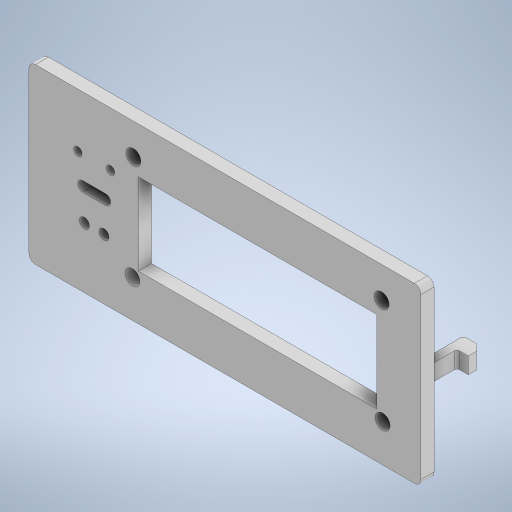
# Autodesk Inventor part: Front
Saved by Autodesk Inventor 2023 (Build 270158000, 158)
## iProperties
Created: 2023-01-08
Part Number: Front
Material: Generisch
Document SubType Name: Modeling
Designer: Benedikt
Density: 1 g/cm^3
Appearance: Vorgabe
Mass: 13.2 g
Surface Area: 108.904 cm^2
Volume: 13.2 cm^3
Author: Benedikt
Autodesk Inventor part; units mm, degrees
ref_plane "YZ Plane" through (0, 0, 0) normal (1, 0, 0) x (0, 1, 0)
ref_plane "XZ Plane" through (0, 0, 0) normal (0, 1, 0) x (-1, 0, 0)
ref_plane "XY Plane" through (0, 0, 0) normal (0, 0, 1) x (1, 0, 0)
sketch "Skizze1" plane through (0, 0, 0) normal (0, 0, 1) x (1, 0, 0)
  line L0 (-60, -26.5) -> (60, -26.5)
  line L1 (60, -26.5) -> (60, 26.5)
  line L2 (60, 26.5) -> (-60, 26.5)
  line L3 (-60, 26.5) -> (-60, -26.5)
  line L4 (-60, -26.5) -> (60, 26.5) construction
  line L5 (60, -26.5) -> (-60, 26.5) construction
  point P0 (0, 0)
  dimension "d0" = 53
  dimension "d1" = 120
  constraints: 12 end point, 2 midpoint, 2 parallel, 1 horizontal, 1 perpendicular
  measures "d0" distance of L0.end L1.end
  measures "d1" distance of L1.end L2.end
extrude "Extrusion1" add sketch "Skizze1" along normal blind 4
sketch "Skizze2" plane through (0, 0, 0) normal (0, 0, -1) x (-1, 0, 0)
  line L0 (-60, -23.5) -> (-60, -26.5) construction
  line L1 (-54, -4) -> (-56.5, -4)
  line L2 (-56.5, -4) -> (-56.5, 1)
  line L3 (-56.5, 1) -> (-54, 1)
  line L4 (-54, 1) -> (-54, -4)
  line L5 (-54, -4) -> (-56.5, 1) construction
  line L6 (-56.5, -4) -> (-54, 1) construction
  line L7 (54, -1) -> (56.5, -1)
  line L8 (56.5, -1) -> (56.5, 4)
  line L9 (56.5, 4) -> (54, 4)
  line L10 (54, 4) -> (54, -1)
  line L11 (54, -1) -> (56.5, 4) construction
  line L12 (56.5, -1) -> (54, 4) construction
  line L13 (60, -26.5) -> (-60, -26.5) projected
  point P0 (0, 0)
  point P1 (-55.25, -1.5)
  point P2 (-55.25, -1.5)
  dimension "d5" = 2.5
  dimension "d6" = 5
  dimension "d68" = 25
  constraints: 26 end point, 2 midpoint, 2 parallel, 1 horizontal, 1 perpendicular
  measures "d5" distance of L2.end L3.end
  measures "d6" distance of L3.end L1.start
  measures "d68" distance from line of L13 point (-55.25, -1.5)
extrude "Extrusion2" add sketch "Skizze2" along normal blind 15 contours L1 L2 L3 L4
sketch "Skizze6" plane through (56.5, -4, 0) normal (1, 0, 0) x (0, 0, -1)
  line L0 (15, 5) -> (15, 0) projected
  line L1 (15, 2.5) -> (0, 2.5)
  line L2 (0, -22.5) -> (0, 30.5) projected
  line L3 (10.5, 0) -> (15, 0)
  line L4 (15, 0) -> (15, 5)
  line L5 (15, 5) -> (10.5, 5)
  line L6 (10.5, 5) -> (10.5, 0)
  line L7 (10.5, 0) -> (15, 5) construction
  line L8 (15, 0) -> (10.5, 5) construction
  point P0 (0, 4)
  point P1 (12.75, 2.5)
  point P2 (15, 0)
  dimension "d19" = 4.5
  dimension "d20" = 5
  constraints: 14 end point, 3 midpoint, 3 point on line, 2 horizontal, 2 parallel, 1 perpendicular
  measures "d19" distance of L4.end L5.end
  measures "d20" distance of L5.end L3.start
extrude "Extrusion5" add sketch "Skizze6" along normal blind 3.5
mirror "Spiegeln2" about plane through (0, 0, 0) normal (1, 0, 0) of "Extrusion2", "Extrusion5"
sketch "Skizze7" plane through (0, 0, 4) normal (0, 0, 1) x (1, 0, 0)
  line L0 (-26.5, -12.5) -> (46.5, -12.5)
  line L1 (46.5, -12.5) -> (46.5, 12.5)
  line L2 (46.5, 12.5) -> (-26.5, 12.5)
  line L3 (-26.5, 12.5) -> (-26.5, -12.5)
  line L4 (-26.5, -12.5) -> (46.5, 12.5) construction
  line L5 (46.5, -12.5) -> (-26.5, 12.5) construction
  point P0 (0, 0)
  point P1 (10, 0)
  dimension "d23" = 10
  dimension "d24" = 73
  dimension "d25" = 25
  constraints: 12 end point, 2 midpoint, 2 parallel, 1 horizontal, 1 perpendicular
  measures "d23" distance of point (10, 0) point (0, 0)
  measures "d24" distance of L2.end L1.end
  measures "d25" distance of L1.end L0.end
extrude "Extrusion6" cut sketch "Skizze7" against normal through all
sketch "Skizze8" plane through (0, 0, 4) normal (0, 0, 1) x (1, 0, 0)
  line L0 (-60, 26.5) -> (-60, -26.5) projected
  line L1 (-60, 0) -> (60, 0)
  line L2 (60, -26.5) -> (60, 26.5) projected
  line L3 (-56, 10) -> (-26.5, 10) construction
  line L4 (-26.5, -12.5) -> (-26.5, 12.5) construction
  circle A0 centre (-45, 10) radius 1.25
  line L5 (-40, 10) -> (-40, 12.8313) construction
  circle A1 centre (-35, 10) radius 1.25
  line L6 (-40, 10) -> (-40, 0) construction
  line L7 (-43.5, 1.5) -> (-36.5, 1.5) construction
  line L8 (-43.5, 0) -> (-36.5, 0)
  line L9 (-36.5, 3) -> (-43.5, 3)
  arc A2 (-43.5, 3) -> (-43.5, 0) centre (-43.5, 1.5) ccw
  arc A3 (-36.5, 0) -> (-36.5, 3) centre (-36.5, 1.5) ccw
  point P0 (0, 0)
  point P1 (-26.5, 0)
  point P2 (-40, 1.5)
  dimension "d28" = 10
  dimension "d29" = 2.5
  dimension "d30" = 10
  dimension "d31" = 7
  dimension "d55" = 13.5
  dimension "d69" = 3
  constraints: 16 end point, 4 centre point, 4 midpoint, 4 point on circle, 4 tangent, 3 point on line, 2 parallel, 2 perpendicular, 1 symmetric about line, 1 vertical, 1 other
  measures "d28" distance of point (-26.5, 0) L3.end
  measures "d29" diameter of A0
  measures "d30" distance of A1.centre A0.centre
  measures "d31" vertical distance of L9.end A0.centre
  measures "d55" distance from line of L4 L5.start
  measures "d69" distance between parallel lines of L9 L8
extrude "Extrusion7" cut sketch "Skizze8" against normal blind 10
sketch "Skizze9" plane through (0, 0, 4) normal (0, 0, 1) x (1, 0, 0)
  circle A0 centre (-28, 17) radius 2.25
  line L0 (-26.5, 12.5) -> (46.5, 12.5) projected
  line L1 (46.5, 12.5) -> (-26.5, 12.5) projected
  line L2 (10, 12.5) -> (10, -12.5)
  line L3 (-25.5, 0) -> (45.5, 0)
  circle A1 centre (48, 17) radius 2.25
  circle A2 centre (-28.3, -15) radius 2.25
  line L4 (46.5, -12.5) -> (-26.5, -12.5) projected
  line L5 (-26.5, -12.5) -> (-26.5, 12.5) projected
  circle A3 centre (48.3, -15) radius 2.25
  point P0 (0, 0)
  dimension "d35" = 4.5
  dimension "d37" = 4.5
  dimension "d40" = 2.5
  dimension "d41" = 1.8
  dimension "d42" = 4.5
  dimension "d53" = 1.5
  constraints: 4 centre point, 4 end point, 2 symmetric about line, 1 horizontal, 1 midpoint, 3 other
  measures "d35" distance from line of L0 A0.centre
  measures "d37" diameter of A0
  measures "d40" distance from line of L4 A2.centre
  measures "d42" diameter of A2
extrude "Extrusion8" cut sketch "Skizze9" against normal blind 10 contours A0 | A1 | A2 | A3
fillet "Rundung1" radius 2 4 edges at (-60, 26.5, 2) (60, 26.5, 2) (-60, -26.5, 2) (60, -26.5, 2)
fillet "Rundung4" radius 0.8 4 edges at (56.5, -1.5, -10.5) (54, -1.5, -15) (-54, -1.5, -15) (-56.5, -1.5, -10.5)
fillet "Rundung5" radius 2 4 edges at (55.25, 1, 0) (55.25, -4, 0) (-55.25, 1, 0) (-55.25, -4, 0)
chamfer "Fase4" distance 2 angle 45 2 edges at (60, -1.5, -15) (-60, -1.5, -15)
sketch "Skizze11" plane through (0, 0, 4) normal (0, 0, 1) x (1, 0, 0)
  line L0 (-36.5, 0) -> (-43.5, 0) construction
  line L1 (-40, 0) -> (-40, -26.5) construction
  line L2 (-58, -26.5) -> (58, -26.5) construction
  circle A0 centre (-43, -8) radius 1.5
  circle A1 centre (-37, -8) radius 1.5
  line L3 (-43, -8) -> (-40, -8) construction
  line L4 (-37, -8) -> (-40, -8) construction
  point P0 (0, 0)
  dimension "d70" = 3
  dimension "d71" = 3
  dimension "d72" = 3
  dimension "d73" = 8
  constraints: 6 end point, 2 centre point, 2 point on line, 1 collinear, 1 horizontal, 1 midpoint, 1 symmetric about line, 1 vertical
  measures "d70" diameter of A0
  measures "d71" diameter of A1
  measures "d73" distance from line of L0 L3.end
extrude "Extrusion10" cut sketch "Skizze11" against normal blind 10
